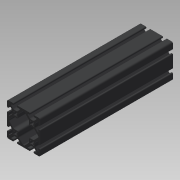
# Autodesk Inventor part: 3030-S
Saved by Autodesk Inventor 2013 (Build 170138000, 138)
## iProperties
Company: 80/20 Inc.
Created: 2014-04-23
Part Number: 3030-S
Material: Generic
Document SubType Name: Modeling
Density: 1 g/cm^3
Vendor: 80/20 Inc.
Engineer: Ross Bowman
Designer: Ross Bowman
Catalog Web Link: 8020.net
Material: 6105-T5 Aluminum
Author: Ross Bowman
Keywords: 80/20 , 8020 , T-Slot , Extrusion
Autodesk Inventor part; units mm, degrees
ref_plane "YZ Plane" through (0, 0, 0) normal (1, 0, 0) x (0, 1, 0)
ref_plane "XZ Plane" through (0, 0, 0) normal (0, 1, 0) x (-1, 0, 0)
ref_plane "XY Plane" through (0, 0, 0) normal (0, 0, 1) x (1, 0, 0)
sketch "Sketch1" plane through (0, 0, 0) normal (0, 0, 1) x (1, 0, 0)
  arc A0 (-14.8044, -16.4102) -> (-16.4102, -14.8044) centre (-15.5149, -15.5149) ccw
  line L0 (-16.0771, -17.6936) -> (-14.8044, -16.4102)
  arc A1 (-16.0771, -20.4064) -> (-16.0771, -17.6936) centre (-19.05, -19.05) ccw
  line L1 (-14.7067, -21.7769) -> (-16.0771, -20.4064)
  arc A2 (-16.3231, -23.3933) -> (-14.7067, -21.7769) centre (-15.5149, -22.5851) ccw
  line L2 (-17.6936, -22.0229) -> (-16.3231, -23.3933)
  arc A3 (-20.4064, -22.0229) -> (-17.6936, -22.0229) centre (-19.05, -19.05) ccw
  line L3 (-21.7769, -23.3933) -> (-20.4064, -22.0229)
  arc A4 (-23.3933, -21.7769) -> (-21.7769, -23.3933) centre (-22.5851, -22.5851) ccw
  line L4 (-22.0229, -20.4064) -> (-23.3933, -21.7769)
  arc A5 (-22.0229, -17.6936) -> (-22.0229, -20.4064) centre (-19.05, -19.05) ccw
  line L5 (-23.3933, -16.3231) -> (-22.0229, -17.6936)
  arc A6 (-21.7769, -14.7067) -> (-23.3933, -16.3231) centre (-22.5851, -15.5149) ccw
  line L6 (-20.4064, -16.0771) -> (-21.7769, -14.7067)
  arc A7 (-17.6936, -16.0771) -> (-20.4064, -16.0771) centre (-19.05, -19.05) ccw
  line L7 (-16.4102, -14.8044) -> (-17.6936, -16.0771)
  arc A8 (-14.8044, 21.6898) -> (-16.4102, 23.2956) centre (-15.5149, 22.5851) ccw
  line L8 (-16.0771, 20.4064) -> (-14.8044, 21.6898)
  arc A9 (-16.0771, 17.6936) -> (-16.0771, 20.4064) centre (-19.05, 19.05) ccw
  line L9 (-14.7067, 16.3231) -> (-16.0771, 17.6936)
  arc A10 (-16.3231, 14.7067) -> (-14.7067, 16.3231) centre (-15.5149, 15.5149) ccw
  line L10 (-17.6936, 16.0771) -> (-16.3231, 14.7067)
  arc A11 (-20.4064, 16.0771) -> (-17.6936, 16.0771) centre (-19.05, 19.05) ccw
  line L11 (-21.7769, 14.7067) -> (-20.4064, 16.0771)
  arc A12 (-23.3933, 16.3231) -> (-21.7769, 14.7067) centre (-22.5851, 15.5149) ccw
  line L12 (-22.0229, 17.6936) -> (-23.3933, 16.3231)
  arc A13 (-22.0229, 20.4064) -> (-22.0229, 17.6936) centre (-19.05, 19.05) ccw
  line L13 (-23.3933, 21.7769) -> (-22.0229, 20.4064)
  arc A14 (-21.7769, 23.3933) -> (-23.3933, 21.7769) centre (-22.5851, 22.5851) ccw
  line L14 (-20.4064, 22.0229) -> (-21.7769, 23.3933)
  arc A15 (-17.6936, 22.0229) -> (-20.4064, 22.0229) centre (-19.05, 19.05) ccw
  line L15 (-16.4102, 23.2956) -> (-17.6936, 22.0229)
  arc A16 (16.4102, -14.8044) -> (14.8044, -16.4102) centre (15.5149, -15.5149) ccw
  line L16 (17.6936, -16.0771) -> (16.4102, -14.8044)
  arc A17 (20.4064, -16.0771) -> (17.6936, -16.0771) centre (19.05, -19.05) ccw
  line L17 (21.7769, -14.7067) -> (20.4064, -16.0771)
  arc A18 (23.3933, -16.3231) -> (21.7769, -14.7067) centre (22.5851, -15.5149) ccw
  line L18 (22.0229, -17.6936) -> (23.3933, -16.3231)
  arc A19 (22.0229, -20.4064) -> (22.0229, -17.6936) centre (19.05, -19.05) ccw
  line L19 (23.3933, -21.7769) -> (22.0229, -20.4064)
  arc A20 (21.7769, -23.3933) -> (23.3933, -21.7769) centre (22.5851, -22.5851) ccw
  line L20 (20.4064, -22.0229) -> (21.7769, -23.3933)
  arc A21 (17.6936, -22.0229) -> (20.4064, -22.0229) centre (19.05, -19.05) ccw
  line L21 (16.3231, -23.3933) -> (17.6936, -22.0229)
  arc A22 (14.7067, -21.7769) -> (16.3231, -23.3933) centre (15.5149, -22.5851) ccw
  line L22 (16.0771, -20.4064) -> (14.7067, -21.7769)
  arc A23 (16.0771, -17.6936) -> (16.0771, -20.4064) centre (19.05, -19.05) ccw
  line L23 (14.8044, -16.4102) -> (16.0771, -17.6936)
  arc A24 (12.1803, 15.3553) -> (15.3553, 12.1803) centre (15.3553, 15.3553) ccw
  line L24 (21.0785, 12.1803) -> (15.3553, 12.1803)
  arc A25 (24.4372, 10.7892) -> (21.0785, 12.1803) centre (21.0785, 7.4305) ccw
  line L25 (33.1609, 2.0655) -> (24.4372, 10.7892)
  arc A26 (33.1609, -2.0655) -> (33.1609, 2.0655) centre (31.0954, 0) ccw
  line L26 (24.4372, -10.7892) -> (33.1609, -2.0655)
  arc A27 (21.0785, -12.1803) -> (24.4372, -10.7892) centre (21.0785, -7.4305) ccw
  line L27 (15.3553, -12.1803) -> (21.0785, -12.1803)
  arc A28 (15.3553, -12.1803) -> (12.1803, -15.3553) centre (15.3553, -15.3553) ccw
  line L28 (12.1803, -21.0785) -> (12.1803, -15.3553)
  arc A29 (10.7892, -24.4372) -> (12.1803, -21.0785) centre (7.4305, -21.0785) ccw
  line L29 (2.0655, -33.1609) -> (10.7892, -24.4372)
  arc A30 (-2.0655, -33.1609) -> (2.0655, -33.1609) centre (0, -31.0954) ccw
  line L30 (-10.7892, -24.4372) -> (-2.0655, -33.1609)
  arc A31 (-12.1803, -21.0785) -> (-10.7892, -24.4372) centre (-7.4305, -21.0785) ccw
  line L31 (-12.1803, -15.3553) -> (-12.1803, -21.0785)
  arc A32 (-12.1803, -15.3553) -> (-15.3553, -12.1803) centre (-15.3553, -15.3553) ccw
  line L32 (-21.0785, -12.1803) -> (-15.3553, -12.1803)
  arc A33 (-24.4372, -10.7892) -> (-21.0785, -12.1803) centre (-21.0785, -7.4305) ccw
  line L33 (-33.1609, -2.0655) -> (-24.4372, -10.7892)
  arc A34 (-33.1609, 2.0655) -> (-33.1609, -2.0655) centre (-31.0954, 0) ccw
  line L34 (-24.4372, 10.7892) -> (-33.1609, 2.0655)
  arc A35 (-21.0785, 12.1803) -> (-24.4372, 10.7892) centre (-21.0785, 7.4305) ccw
  line L35 (-15.3553, 12.1803) -> (-21.0785, 12.1803)
  arc A36 (-15.3553, 12.1803) -> (-12.1803, 15.3553) centre (-15.3553, 15.3553) ccw
  line L36 (-12.1803, 21.0785) -> (-12.1803, 15.3553)
  arc A37 (-10.7892, 24.4372) -> (-12.1803, 21.0785) centre (-7.4305, 21.0785) ccw
  line L37 (-2.0655, 33.1609) -> (-10.7892, 24.4372)
  arc A38 (2.0655, 33.1609) -> (-2.0655, 33.1609) centre (0, 31.0954) ccw
  line L38 (10.7892, 24.4372) -> (2.0655, 33.1609)
  arc A39 (12.1803, 21.0785) -> (10.7892, 24.4372) centre (7.4305, 21.0785) ccw
  line L39 (12.1803, 15.3553) -> (12.1803, 21.0785)
  arc A40 (16.4102, 23.2956) -> (14.8044, 21.6898) centre (15.5149, 22.5851) ccw
  line L40 (17.6936, 22.0229) -> (16.4102, 23.2956)
  arc A41 (20.4064, 22.0229) -> (17.6936, 22.0229) centre (19.05, 19.05) ccw
  line L41 (21.7769, 23.3933) -> (20.4064, 22.0229)
  arc A42 (23.3933, 21.7769) -> (21.7769, 23.3933) centre (22.5851, 22.5851) ccw
  line L42 (22.0229, 20.4064) -> (23.3933, 21.7769)
  arc A43 (22.0229, 17.6936) -> (22.0229, 20.4064) centre (19.05, 19.05) ccw
  line L43 (23.3933, 16.3231) -> (22.0229, 17.6936)
  arc A44 (21.7769, 14.7067) -> (23.3933, 16.3231) centre (22.5851, 15.5149) ccw
  line L44 (20.4064, 16.0771) -> (21.7769, 14.7067)
  arc A45 (17.6936, 16.0771) -> (20.4064, 16.0771) centre (19.05, 19.05) ccw
  line L45 (16.3231, 14.7067) -> (17.6936, 16.0771)
  arc A46 (14.7067, 16.3231) -> (16.3231, 14.7067) centre (15.5149, 15.5149) ccw
  line L46 (16.0771, 17.6936) -> (14.7067, 16.3231)
  arc A47 (16.0771, 20.4064) -> (16.0771, 17.6936) centre (19.05, 19.05) ccw
  line L47 (14.8044, 21.6898) -> (16.0771, 20.4064)
  arc A48 (14.986, 36.5252) -> (13.4112, 38.1) centre (13.4112, 36.5252) ccw
  line L48 (13.4112, 38.1) -> (-13.4112, 38.1)
  arc A49 (-13.4112, 38.1) -> (-14.986, 36.5252) centre (-13.4112, 36.5252) ccw
  line L49 (-14.986, 36.5252) -> (-14.986, 35.6108)
  arc A50 (-14.986, 35.6108) -> (-13.4112, 34.036) centre (-13.4112, 35.6108) ccw
  line L50 (-13.4112, 34.036) -> (-9.652, 34.036)
  arc A51 (-8.763, 33.147) -> (-9.652, 34.036) centre (-9.652, 33.147) ccw
  line L51 (-8.763, 33.147) -> (-8.763, 32.5789)
  arc A52 (-9.0234, 31.9503) -> (-8.763, 32.5789) centre (-9.652, 32.5789) ccw
  line L52 (-9.0234, 31.9503) -> (-13.6628, 27.3108)
  arc A53 (-17.0215, 25.9197) -> (-13.6628, 27.3108) centre (-17.0215, 30.6695) ccw
  line L53 (-17.0215, 25.9197) -> (-21.0785, 25.9197)
  arc A54 (-24.4372, 27.3108) -> (-21.0785, 25.9197) centre (-21.0785, 30.6695) ccw
  line L54 (-24.4372, 27.3108) -> (-29.0766, 31.9503)
  arc A55 (-29.337, 32.5789) -> (-29.0766, 31.9503) centre (-28.448, 32.5789) ccw
  line L55 (-29.337, 32.5789) -> (-29.337, 33.147)
  arc A56 (-28.448, 34.036) -> (-29.337, 33.147) centre (-28.448, 33.147) ccw
  line L56 (-28.448, 34.036) -> (-24.6888, 34.036)
  arc A57 (-24.6888, 34.036) -> (-23.114, 35.6108) centre (-24.6888, 35.6108) ccw
  line L57 (-23.114, 35.6108) -> (-23.114, 36.5252)
  arc A58 (-23.114, 36.5252) -> (-24.6888, 38.1) centre (-24.6888, 36.5252) ccw
  line L58 (-24.6888, 38.1) -> (-34.925, 38.1)
  arc A59 (-34.925, 38.1) -> (-38.1, 34.925) centre (-34.925, 34.925) ccw
  line L59 (-38.1, 34.925) -> (-38.1, 24.6888)
  arc A60 (-38.1, 24.6888) -> (-36.5252, 23.114) centre (-36.5252, 24.6888) ccw
  line L60 (-36.5252, 23.114) -> (-35.6108, 23.114)
  arc A61 (-35.6108, 23.114) -> (-34.036, 24.6888) centre (-35.6108, 24.6888) ccw
  line L61 (-34.036, 24.6888) -> (-34.036, 28.448)
  arc A62 (-33.147, 29.337) -> (-34.036, 28.448) centre (-33.147, 28.448) ccw
  line L62 (-33.147, 29.337) -> (-32.5789, 29.337)
  arc A63 (-31.9503, 29.0766) -> (-32.5789, 29.337) centre (-32.5789, 28.448) ccw
  line L63 (-31.9503, 29.0766) -> (-27.3108, 24.4372)
  arc A64 (-25.9197, 21.0785) -> (-27.3108, 24.4372) centre (-30.6695, 21.0785) ccw
  line L64 (-25.9197, 21.0785) -> (-25.9197, 17.0215)
  arc A65 (-27.3108, 13.6628) -> (-25.9197, 17.0215) centre (-30.6695, 17.0215) ccw
  line L65 (-27.3108, 13.6628) -> (-31.9503, 9.0234)
  arc A66 (-32.5789, 8.763) -> (-31.9503, 9.0234) centre (-32.5789, 9.652) ccw
  line L66 (-32.5789, 8.763) -> (-33.147, 8.763)
  arc A67 (-34.036, 9.652) -> (-33.147, 8.763) centre (-33.147, 9.652) ccw
  line L67 (-34.036, 9.652) -> (-34.036, 13.4112)
  arc A68 (-34.036, 13.4112) -> (-35.6108, 14.986) centre (-35.6108, 13.4112) ccw
  line L68 (-35.6108, 14.986) -> (-36.5252, 14.986)
  arc A69 (-36.5252, 14.986) -> (-38.1, 13.4112) centre (-36.5252, 13.4112) ccw
  line L69 (-38.1, 13.4112) -> (-38.1, -13.4112)
  arc A70 (-38.1, -13.4112) -> (-36.5252, -14.986) centre (-36.5252, -13.4112) ccw
  line L70 (-36.5252, -14.986) -> (-35.6108, -14.986)
  arc A71 (-35.6108, -14.986) -> (-34.036, -13.4112) centre (-35.6108, -13.4112) ccw
  line L71 (-34.036, -13.4112) -> (-34.036, -9.652)
  arc A72 (-33.147, -8.763) -> (-34.036, -9.652) centre (-33.147, -9.652) ccw
  line L72 (-33.147, -8.763) -> (-32.5789, -8.763)
  arc A73 (-31.9503, -9.0234) -> (-32.5789, -8.763) centre (-32.5789, -9.652) ccw
  line L73 (-31.9503, -9.0234) -> (-27.3108, -13.6628)
  arc A74 (-25.9197, -17.0215) -> (-27.3108, -13.6628) centre (-30.6695, -17.0215) ccw
  line L74 (-25.9197, -17.0215) -> (-25.9197, -21.0785)
  arc A75 (-27.3108, -24.4372) -> (-25.9197, -21.0785) centre (-30.6695, -21.0785) ccw
  line L75 (-27.3108, -24.4372) -> (-31.9503, -29.0766)
  arc A76 (-32.5789, -29.337) -> (-31.9503, -29.0766) centre (-32.5789, -28.448) ccw
  line L76 (-32.5789, -29.337) -> (-33.147, -29.337)
  arc A77 (-34.036, -28.448) -> (-33.147, -29.337) centre (-33.147, -28.448) ccw
  line L77 (-34.036, -28.448) -> (-34.036, -24.6888)
  arc A78 (-34.036, -24.6888) -> (-35.6108, -23.114) centre (-35.6108, -24.6888) ccw
  line L78 (-35.6108, -23.114) -> (-36.5252, -23.114)
  arc A79 (-36.5252, -23.114) -> (-38.1, -24.6888) centre (-36.5252, -24.6888) ccw
  line L79 (-38.1, -24.6888) -> (-38.1, -34.925)
  arc A80 (-38.1, -34.925) -> (-34.925, -38.1) centre (-34.925, -34.925) ccw
  line L80 (-34.925, -38.1) -> (-24.6888, -38.1)
  arc A81 (-24.6888, -38.1) -> (-23.114, -36.5252) centre (-24.6888, -36.5252) ccw
  line L81 (-23.114, -36.5252) -> (-23.114, -35.6108)
  arc A82 (-23.114, -35.6108) -> (-24.6888, -34.036) centre (-24.6888, -35.6108) ccw
  line L82 (-24.6888, -34.036) -> (-28.448, -34.036)
  arc A83 (-29.337, -33.147) -> (-28.448, -34.036) centre (-28.448, -33.147) ccw
  line L83 (-29.337, -33.147) -> (-29.337, -32.5789)
  arc A84 (-29.0766, -31.9503) -> (-29.337, -32.5789) centre (-28.448, -32.5789) ccw
  line L84 (-29.0766, -31.9503) -> (-24.4372, -27.3108)
  arc A85 (-21.0785, -25.9197) -> (-24.4372, -27.3108) centre (-21.0785, -30.6695) ccw
  line L85 (-21.0785, -25.9197) -> (-17.0215, -25.9197)
  arc A86 (-13.6628, -27.3108) -> (-17.0215, -25.9197) centre (-17.0215, -30.6695) ccw
  line L86 (-13.6628, -27.3108) -> (-9.0234, -31.9503)
  arc A87 (-8.763, -32.5789) -> (-9.0234, -31.9503) centre (-9.652, -32.5789) ccw
  line L87 (-8.763, -32.5789) -> (-8.763, -33.147)
  arc A88 (-9.652, -34.036) -> (-8.763, -33.147) centre (-9.652, -33.147) ccw
  line L88 (-9.652, -34.036) -> (-13.4112, -34.036)
  arc A89 (-13.4112, -34.036) -> (-14.986, -35.6108) centre (-13.4112, -35.6108) ccw
  line L89 (-14.986, -35.6108) -> (-14.986, -36.5252)
  arc A90 (-14.986, -36.5252) -> (-13.4112, -38.1) centre (-13.4112, -36.5252) ccw
  line L90 (-13.4112, -38.1) -> (13.4112, -38.1)
  arc A91 (13.4112, -38.1) -> (14.986, -36.5252) centre (13.4112, -36.5252) ccw
  line L91 (14.986, -36.5252) -> (14.986, -35.6108)
  arc A92 (14.986, -35.6108) -> (13.4112, -34.036) centre (13.4112, -35.6108) ccw
  line L92 (13.4112, -34.036) -> (9.652, -34.036)
  arc A93 (8.763, -33.147) -> (9.652, -34.036) centre (9.652, -33.147) ccw
  line L93 (8.763, -33.147) -> (8.763, -32.5789)
  arc A94 (9.0234, -31.9503) -> (8.763, -32.5789) centre (9.652, -32.5789) ccw
  line L94 (9.0234, -31.9503) -> (13.6628, -27.3108)
  arc A95 (17.0215, -25.9197) -> (13.6628, -27.3108) centre (17.0215, -30.6695) ccw
  line L95 (17.0215, -25.9197) -> (21.0785, -25.9197)
  arc A96 (24.4372, -27.3108) -> (21.0785, -25.9197) centre (21.0785, -30.6695) ccw
  line L96 (24.4372, -27.3108) -> (29.0766, -31.9503)
  arc A97 (29.337, -32.5789) -> (29.0766, -31.9503) centre (28.448, -32.5789) ccw
  line L97 (29.337, -32.5789) -> (29.337, -33.147)
  arc A98 (28.448, -34.036) -> (29.337, -33.147) centre (28.448, -33.147) ccw
  line L98 (28.448, -34.036) -> (24.6888, -34.036)
  arc A99 (24.6888, -34.036) -> (23.114, -35.6108) centre (24.6888, -35.6108) ccw
  line L99 (23.114, -35.6108) -> (23.114, -36.5252)
  arc A100 (23.114, -36.5252) -> (24.6888, -38.1) centre (24.6888, -36.5252) ccw
  line L100 (24.6888, -38.1) -> (34.925, -38.1)
  arc A101 (34.925, -38.1) -> (38.1, -34.925) centre (34.925, -34.925) ccw
  line L101 (38.1, -34.925) -> (38.1, -24.6888)
  arc A102 (38.1, -24.6888) -> (36.5252, -23.114) centre (36.5252, -24.6888) ccw
  line L102 (36.5252, -23.114) -> (35.6108, -23.114)
  arc A103 (35.6108, -23.114) -> (34.036, -24.6888) centre (35.6108, -24.6888) ccw
  line L103 (34.036, -24.6888) -> (34.036, -28.448)
  arc A104 (33.147, -29.337) -> (34.036, -28.448) centre (33.147, -28.448) ccw
  line L104 (33.147, -29.337) -> (32.5789, -29.337)
  arc A105 (31.9503, -29.0766) -> (32.5789, -29.337) centre (32.5789, -28.448) ccw
  line L105 (31.9503, -29.0766) -> (27.3108, -24.4372)
  arc A106 (25.9197, -21.0785) -> (27.3108, -24.4372) centre (30.6695, -21.0785) ccw
  line L106 (25.9197, -21.0785) -> (25.9197, -17.0215)
  arc A107 (27.3108, -13.6628) -> (25.9197, -17.0215) centre (30.6695, -17.0215) ccw
  line L107 (27.3108, -13.6628) -> (31.9503, -9.0234)
  arc A108 (32.5789, -8.763) -> (31.9503, -9.0234) centre (32.5789, -9.652) ccw
  line L108 (32.5789, -8.763) -> (33.147, -8.763)
  arc A109 (34.036, -9.652) -> (33.147, -8.763) centre (33.147, -9.652) ccw
  line L109 (34.036, -9.652) -> (34.036, -13.4112)
  arc A110 (34.036, -13.4112) -> (35.6108, -14.986) centre (35.6108, -13.4112) ccw
  line L110 (35.6108, -14.986) -> (36.5252, -14.986)
  arc A111 (36.5252, -14.986) -> (38.1, -13.4112) centre (36.5252, -13.4112) ccw
  line L111 (38.1, -13.4112) -> (38.1, 13.4112)
  arc A112 (38.1, 13.4112) -> (36.5252, 14.986) centre (36.5252, 13.4112) ccw
  line L112 (36.5252, 14.986) -> (35.6108, 14.986)
  arc A113 (35.6108, 14.986) -> (34.036, 13.4112) centre (35.6108, 13.4112) ccw
  line L113 (34.036, 13.4112) -> (34.036, 9.652)
  arc A114 (33.147, 8.763) -> (34.036, 9.652) centre (33.147, 9.652) ccw
  line L114 (33.147, 8.763) -> (32.5789, 8.763)
  arc A115 (31.9503, 9.0234) -> (32.5789, 8.763) centre (32.5789, 9.652) ccw
  line L115 (31.9503, 9.0234) -> (27.3108, 13.6628)
  arc A116 (25.9197, 17.0215) -> (27.3108, 13.6628) centre (30.6695, 17.0215) ccw
  line L116 (25.9197, 17.0215) -> (25.9197, 21.0785)
  arc A117 (27.3108, 24.4372) -> (25.9197, 21.0785) centre (30.6695, 21.0785) ccw
  line L117 (27.3108, 24.4372) -> (31.9503, 29.0766)
  arc A118 (32.5789, 29.337) -> (31.9503, 29.0766) centre (32.5789, 28.448) ccw
  line L118 (32.5789, 29.337) -> (33.147, 29.337)
  arc A119 (34.036, 28.448) -> (33.147, 29.337) centre (33.147, 28.448) ccw
  line L119 (34.036, 28.448) -> (34.036, 24.6888)
  arc A120 (34.036, 24.6888) -> (35.6108, 23.114) centre (35.6108, 24.6888) ccw
  line L120 (35.6108, 23.114) -> (36.5252, 23.114)
  arc A121 (36.5252, 23.114) -> (38.1, 24.6888) centre (36.5252, 24.6888) ccw
  line L121 (38.1, 24.6888) -> (38.1, 34.925)
  arc A122 (38.1, 34.925) -> (34.925, 38.1) centre (34.925, 34.925) ccw
  line L122 (34.925, 38.1) -> (24.6888, 38.1)
  arc A123 (24.6888, 38.1) -> (23.114, 36.5252) centre (24.6888, 36.5252) ccw
  line L123 (23.114, 36.5252) -> (23.114, 35.6108)
  arc A124 (23.114, 35.6108) -> (24.6888, 34.036) centre (24.6888, 35.6108) ccw
  line L124 (24.6888, 34.036) -> (28.448, 34.036)
  arc A125 (29.337, 33.147) -> (28.448, 34.036) centre (28.448, 33.147) ccw
  line L125 (29.337, 33.147) -> (29.337, 32.5789)
  arc A126 (29.0766, 31.9503) -> (29.337, 32.5789) centre (28.448, 32.5789) ccw
  line L126 (29.0766, 31.9503) -> (24.4372, 27.3108)
  arc A127 (21.0785, 25.9197) -> (24.4372, 27.3108) centre (21.0785, 30.6695) ccw
  line L127 (21.0785, 25.9197) -> (17.0215, 25.9197)
  arc A128 (13.6628, 27.3108) -> (17.0215, 25.9197) centre (17.0215, 30.6695) ccw
  line L128 (13.6628, 27.3108) -> (9.0234, 31.9503)
  arc A129 (8.763, 32.5789) -> (9.0234, 31.9503) centre (9.652, 32.5789) ccw
  line L129 (8.763, 32.5789) -> (8.763, 33.147)
  arc A130 (9.652, 34.036) -> (8.763, 33.147) centre (9.652, 33.147) ccw
  line L130 (9.652, 34.036) -> (13.4112, 34.036)
  arc A131 (13.4112, 34.036) -> (14.986, 35.6108) centre (13.4112, 35.6108) ccw
  line L131 (14.986, 35.6108) -> (14.986, 36.5252)
  point P0 (0, 0)
  constraints: 264 end point, 264 point on circle, 132 centre point
extrude "Extrusion1" add sketch "Sketch1" against normal blind 304.8
body "Solid1"
